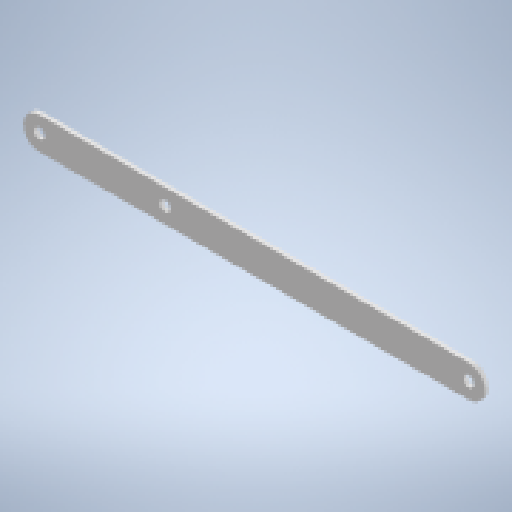
# Autodesk Inventor part: ArmConnector1
Saved by Autodesk Inventor 2024 (Build 280153000, 153)
## iProperties
Created: 2019-01-19
Part Number: ArmConnector1
Material: Generic
Document SubType Name: Modeling
Designer: Teacher
Density: 1 g/cm^3
Appearance: Default
Author: Teacher
Autodesk Inventor part; units mm, degrees
ref_plane "YZ Plane" through (0, 0, 0) normal (1, 0, 0) x (0, 1, 0)
ref_plane "XZ Plane" through (0, 0, 0) normal (0, 1, 0) x (-1, 0, 0)
ref_plane "XY Plane" through (0, 0, 0) normal (0, 0, 1) x (1, 0, 0)
sketch "Sketch1" plane through (0, 0, 0) normal (0, 0, 1) x (1, 0, 0)
  arc A0 (0, -9.7409) -> (0, 9.7409) centre (0, 0) ccw
  arc A1 (-260.35, 9.7409) -> (-260.35, -9.7409) centre (-260.35, 0) ccw
  line L0 (-260.35, 9.7409) -> (0, 9.7409)
  line L1 (0, -9.7409) -> (-260.35, -9.7409)
  circle A2 centre (-260.35, 0) radius 3.2512
  circle A3 centre (0, 0) radius 3.2512
  circle A4 centre (-171.45, 0) radius 3.2512
  dimension "d0" = 19.4818
  dimension "d1" = 19.4818
  dimension "d2" = 260.35
  dimension "d3" = 6.5024
  dimension "d4" = 6.5024
  dimension "d12" = 6.5024
  dimension "d13" = 9.7409
  dimension "d14" = 88.9
  constraints: 5 centre point, 4 end point, 4 point on circle, 3 coincident, 2 tangent, 1 horizontal, 1 horizontal alignment, 1 parallel
  measures "d0" diameter of A0
  measures "d1" diameter of A1
  measures "d2" distance of point (0, 0) A1.centre
  measures "d3" diameter of A2
  measures "d4" diameter of A3
  measures "d12" diameter of A4
  measures "d13" distance from line of L1 A4.centre
  measures "d14" distance of A1.centre A4.centre
extrude "Extrusion1" add sketch "Sketch1" along normal blind 2.54 contours L1 A1 L0 A0 | A4
sketch "Sketch2" plane through (0, 0, 0) normal (0, 0, -1) x (-1, 0, 0)
  circle A0 centre (184.15, 0) radius 3.175
  circle A1 centre (260.35, 0) radius 3.2512 projected
  circle A2 centre (0, 0) radius 3.2512 projected
  line L0 (260.35, 9.7409) -> (0, 9.7409) projected
  arc A3 (0, 9.7409) -> (0, -9.7409) centre (0, 0) ccw projected
  line L1 (0, -9.7409) -> (260.35, -9.7409) projected
  arc A4 (260.35, -9.7409) -> (260.35, 9.7409) centre (260.35, 0) ccw projected
  point P0 (130.175, 9.7409)
  dimension "d7" = 6.35
  dimension "d11" = 76.2
  constraints: 1 centre point, 1 horizontal alignment, 1 midpoint
  measures "d7" diameter of A0
  measures "d11" distance of A0.centre A1.centre
extrude "Extrusion2" cut sketch "Sketch2" against normal through all contours A0
equation "\"d0\" = d1"
body "Solid1"
